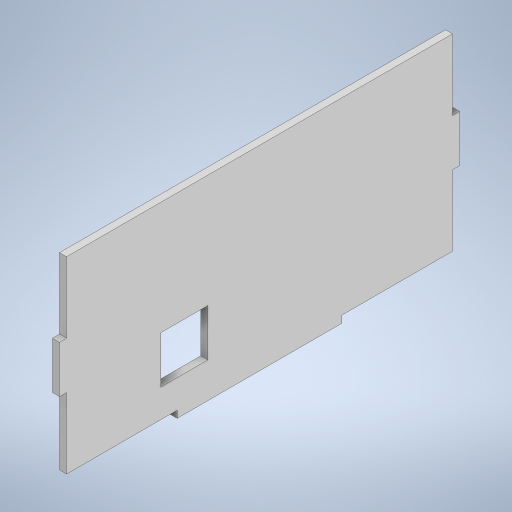
# Autodesk Inventor part: Kiri
Saved by Autodesk Inventor 2024 (Build 280153000, 153)
## iProperties
Created: 2023-08-09
Part Number: Kiri
Material: Generic
Document SubType Name: Modeling
Designer: Asus
Density: 1 g/cm^3
Appearance: Default
Author: Asus
Autodesk Inventor part; units mm, degrees
ref_plane "YZ Plane" through (0, 0, 0) normal (1, 0, 0) x (0, 1, 0)
ref_plane "XZ Plane" through (0, 0, 0) normal (0, 1, 0) x (-1, 0, 0)
ref_plane "XY Plane" through (0, 0, 0) normal (0, 0, 1) x (1, 0, 0)
sketch "Sketch2" plane through (0, 0, 0) normal (1, 0, 0) x (0, 1, 0)
  line L0 (0, 0) -> (3, 0) construction
  line L1 (3, -3) -> (3, -50)
  line L2 (3, -50) -> (0, -50)
  line L3 (0, -50) -> (0, -120)
  line L4 (0, -120) -> (3, -120)
  line L5 (53, 0) -> (53, -3)
  line L6 (33, -3) -> (33, 0)
  line L7 (0, 0) -> (0, -43) construction
  line L8 (0, -43) -> (15, -43) construction
  line L9 (15, -43) -> (35, -43) construction
  line L10 (15, -43) -> (15, -63)
  line L11 (15, -63) -> (35, -63)
  line L12 (35, -63) -> (35, -43)
  line L13 (35, -43) -> (15, -43)
  line L14 (83, -164) -> (83, -117)
  line L15 (3, -167) -> (3, -120)
  line L16 (3, -167) -> (33, -167)
  line L17 (33, -167) -> (33, -170)
  line L18 (33, -170) -> (53, -170)
  line L19 (53, -170) -> (53, -167)
  line L20 (53, -167) -> (83, -167)
  line L21 (83, -167) -> (83, -164)
  line L22 (53, -3) -> (83, -3)
  line L23 (53, 0) -> (33, 0)
  line L24 (33, -3) -> (3, -3)
  line L25 (83, -3) -> (83, -117)
  dimension "d0" = 3
  dimension "d1" = 3
  dimension "d2" = 47
  dimension "d3" = 70
  dimension "d11" = 3
  dimension "d12" = 20
  dimension "d15" = 43
  dimension "d16" = 15
  dimension "d17" = 20
  dimension "d18" = 20
  dimension "d19" = 47
  dimension "d20" = 30
  dimension "d21" = 3
  dimension "d22" = 20
  constraints: 52 end point, 10 perpendicular, 5 point on line, 3 parallel, 3 vertical, 2 horizontal, 1 collinear
  measures "d0" distance of L0.start L0.end
  measures "d1" distance of L0.end L1.start
  measures "d2" distance of L1.start L1.end
  measures "d3" distance of L2.end L3.end
  measures "d11" distance of L5.start L5.end
  measures "d12" distance of L5.end L6.start
  measures "d15" distance of L0.start L7.end
  measures "d16" distance of L7.end L8.end
  measures "d17" distance of L8.end L9.end
  measures "d18" distance of L8.end L10.end
  measures "d19" distance of L15.start L4.end
  measures "d20" distance of L15.start L16.end
  measures "d21" distance of L16.end L17.end
  measures "d22" distance of L17.end L18.end
extrude "Extrusion1" add sketch "Sketch2" along normal blind 3
body "Solid1"
